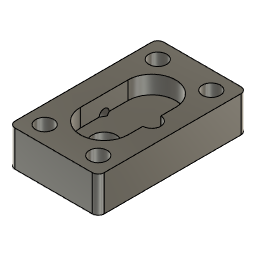
Gear Pump Body v1 (Autodesk Fusion 360 design; units mm, degrees)
Autodesk Fusion 360 part; units mm, degrees
sketch "Sketch1" plane through (0, 0, 0) normal (0, 0, 1) x (1, 0, 0)
  line L0 (0, 0) -> (15, 0)
  line L1 (15, 0) -> (15, 25)
  line L2 (15, 25) -> (0, 25)
  line L3 (0, 25) -> (0, 0)
  circle A0 centre (3, 22) radius 1.5
  circle A1 centre (12, 3) radius 1.5
  circle A2 centre (12, 22) radius 1.5
  circle A3 centre (3, 3) radius 1.5
  line L4 (7.5, 25) -> (7.5, 0) construction
  line L5 (7.5, 12.5) -> (11.5, 12.5) construction
  circle A4 centre (11.5, 12.5) radius 2.5
  dimension "d11" = 15
  dimension "d12" = 25
  dimension "d13" = 3
  dimension "d14" = 3
  dimension "d15" = 3
  dimension "d16" = 3
  dimension "d17" = 3
  dimension "d18" = 3
  dimension "d19" = 3
  dimension "d20" = 3
  dimension "d21" = 3
  dimension "d22" = 3
  dimension "d23" = 3
  dimension "d24" = 3
  dimension "d27" = 4
  dimension "d28" = 5
  constraint horizontal L0
  constraint vertical L1
  constraint horizontal L2
  constraint vertical L3
  constraint coincident L0.start L3.end
  constraint midpoint L2 L4.start
  constraint midpoint L0 L4.end
  constraint midpoint L4 L5.start
  constraint perpendicular L4 L5
  constraint coincident L5.end A4.centre
  measures "d11" distance of L0.start L0.end
  measures "d12" distance of L0.start L2.end
  measures "d13" diameter of A0
  measures "d14" diameter of A1
  measures "d15" diameter of A2
  measures "d16" diameter of A3
  measures "d17" distance of L1 A1.centre
  measures "d18" distance of L3 A3.centre
  measures "d19" distance of L3 A0.centre
  measures "d20" distance of L1 A2.centre
  measures "d21" distance of L2 A2.centre
  measures "d22" distance of L2 A0.centre
  measures "d23" distance of L0 A1.centre
  measures "d24" distance of L0 A3.centre
  measures "d27" distance of L5.start L5.end
  measures "d28" diameter of A4
extrude "Extrude1" add sketch "Sketch1" along normal blind 3
sketch "Sketch2" plane through (0, 0, 3) normal (0, 0, 1) x (-1, 0, 0)
  circle A0 centre (-12, -22) radius 1.5
  circle A1 centre (-12, -3) radius 1.5
  circle A2 centre (-3, -22) radius 1.5
  circle A3 centre (-3, -3) radius 1.5
  circle A4 centre (-11.5, -12.5) radius 2.5
  line L0 (0, -25) -> (0, 0)
  line L1 (0, 0) -> (-15, 0)
  line L2 (-15, 0) -> (-15, -25)
  line L3 (-15, -25) -> (0, -25)
  circle A5 centre (-3, -22) radius 1.5
  circle A6 centre (-12, -22) radius 1.5
  circle A7 centre (-12, -3) radius 1.5
  circle A8 centre (-3, -3) radius 1.5
  line L4 (-7.5, -25) -> (-7.5, 0) construction
  line L5 (0, -12.5) -> (-15, -12.5) construction
  line L6 (-11.5, -16.5) -> (-11.5, -8.5)
  line L7 (-3.5, -8.5) -> (-3.5, -16.5)
  arc A9 (-11.5, -16.5) -> (-3.5, -16.5) centre (-7.5, -16.5) ccw
  arc A10 (-3.5, -8.5) -> (-11.5, -8.5) centre (-7.5, -8.5) ccw
  line L8 (-11.5, -12.5) -> (-3.5, -12.5) construction
  arc A11 (-11.5, -11) -> (-11.5, -14) centre (-11.5, -12.5) ccw
  circle A12 centre (-7.5, -8.5) radius 2
  dimension "d31" = 3
  dimension "d32" = 3
  dimension "d33" = 3
  dimension "d34" = 3
  dimension "d35" = 8
  dimension "d36" = 8
  dimension "d37" = 8
  dimension "d39" = 3
  dimension "d40" = 4
  constraint concentric A2 A5
  constraint concentric A0 A6
  constraint concentric A1 A7
  constraint concentric A3 A8
  constraint midpoint L3 L4.start
  constraint midpoint L1 L4.end
  constraint midpoint L0 L5.start
  constraint midpoint L2 L5.end
  constraint coincident L4 A9.centre
  constraint coincident L4 A10.centre
  constraint vertical L6
  constraint vertical L7
  constraint tangent L7 A9
  constraint tangent L6 A10
  constraint midpoint L6 A4.centre
  constraint midpoint L7 L8.end
  constraint perpendicular L7 L8
  constraint midpoint L5 L8
  constraint coincident A4.centre L8.start
  constraint coincident L6 A11.end
  constraint coincident L6 A11.start
  constraint concentric A10 A12
  measures "d31" diameter of A5
  measures "d32" diameter of A6
  measures "d33" diameter of A7
  measures "d34" diameter of A8
  measures "d35" diameter of A9
  measures "d36" diameter of A10
  measures "d37" distance of A9.centre A10.centre
  measures "d39" diameter of A11
  measures "d40" diameter of A12
extrude "Extrude2" add sketch "Sketch2" along normal blind 3 contours A4 L6 A11 | L0 L1 L2 L3
extrude "Extrude3" cut sketch "Sketch2" against normal blind 1.5 contours A12
fillet "Fillet1" radius 1 4 edges at (15, 0, 3) (0, 0, 3) (0, 25, 3) (15, 25, 3)
sketch "Sketch3" plane through (0, 0, 0) normal (-1, 0, 0) x (0, -1, 0)
  line L0 (-24, 6) -> (-24, 0)
  line L1 (-24, 0) -> (-1, 0)
  line L2 (-1, 0) -> (-1, 6)
  line L3 (-1, 6) -> (-24, 6)
  line L4 (-25, 0) -> (-25, 6)
  line L5 (0, 0) -> (0, 6)
  line L6 (-25, 3) -> (0, 3) construction
  line L7 (-12.5, 6) -> (-12.5, 0) construction
  circle A0 centre (-12.5, 3) radius 2.5
  circle A1 centre (-12.5, 3) radius 1.5
  point P0 (-12.5, 0)
  dimension "d50" = 5
  dimension "d51" = 3
  constraint midpoint L4 L6.start
  constraint midpoint L5 L6.end
  constraint midpoint L3 L7.start
  constraint coincident P0 L7.end
  constraint midpoint L6 A0.centre
  constraint concentric A0 A1
  measures "d50" diameter of A0
  measures "d51" diameter of A1
extrude "Extrude4" cut sketch "Sketch3" against normal blind 1.5 contours A0
extrude "Extrude5" cut sketch "Sketch3" against normal blind 3 contours A1
hole "Hole1" at (3, 12.5, 3) direction (1, 0, 0) diameter 3 depth 0.1 tip angle 118
equation "outer_filet_radius = 1 mm"
equation "mount_hole_diameter = 3 mm"
equation "mount_hole_length_inset = 3 mm"
equation "mount_hole_width_inset = 3 mm"
equation "bottom_thru_hole_diameter = 5 mm"
equation "bottom_plate_depth = 3 mm"
equation "bottom_plate_partial_hole_radius = 4 mm"
equation "bottom_plate_partial_hole_depth = 4.5 mm"
equation "width = 15 mm"
equation "length = 25 mm"
equation "d11 = width"
equation "d12 = length"
equation "d13 = mount_hole_diameter"
equation "d14 = mount_hole_diameter"
equation "d15 = mount_hole_diameter"
equation "d16 = mount_hole_diameter"
equation "d17 = mount_hole_width_inset"
equation "d18 = mount_hole_width_inset"
equation "d19 = mount_hole_width_inset"
equation "d20 = mount_hole_width_inset"
equation "d21 = mount_hole_length_inset"
equation "d22 = mount_hole_length_inset"
equation "d23 = mount_hole_length_inset"
equation "d24 = mount_hole_length_inset"
equation "slot_radius = 4 mm"
equation "slot_length = 16 mm"
equation "d27 = slot_radius"
equation "d28 = bottom_thru_hole_diameter"
equation "d29 = bottom_plate_depth"
equation "d31 = mount_hole_diameter"
equation "d32 = mount_hole_diameter"
equation "d33 = mount_hole_diameter"
equation "d34 = mount_hole_diameter"
equation "d35 = slot_radius * 2"
equation "d36 = slot_radius * 2"
equation "d37 = slot_length - ( slot_radius * 2 )"
equation "slotted_circle_diameter = 3 mm"
equation "d39 = slotted_circle_diameter"
equation "d40 = bottom_plate_partial_hole_radius"
equation "top_plate_thickness = 3 mm"
equation "d42 = top_plate_thickness"
equation "d44 = top_plate_thickness - bottom_plate_partial_hole_depth"
equation "d47 = outer_filet_radius"
equation "outer_side_hole_diameter = 5 mm"
equation "inner_side_hole_diameter = 3 mm"
equation "d50 = outer_side_hole_diameter"
equation "d51 = inner_side_hole_diameter"
equation "outer_side_hole_depth = 1.5 mm"
equation "inner_side_hole_depth = 3 mm"
equation "d54 = -outer_side_hole_depth"
equation "d56 = -inner_side_hole_depth"
